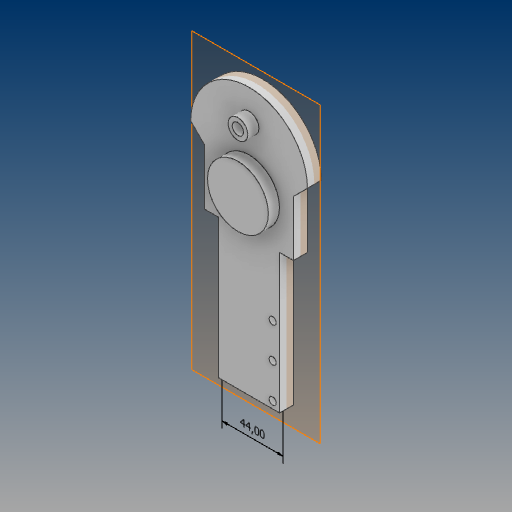
# Autodesk Inventor part: 17_Khau_noi_tiep_cuoi
Saved by Autodesk Inventor 2021 (Build 250183000, 183)
## iProperties
Created: 2024-04-05
Part Number: 17_Khau_noi_tiep_cuoi
Material: Generic
Document SubType Name: Modeling
Designer: Admin
Density: 1 g/cm^3
Appearance: Default
Author: Admin
Autodesk Inventor part; units mm, degrees
ref_plane "YZ Plane" through (0, 0, 0) normal (1, 0, 0) x (0, 1, 0)
ref_plane "XZ Plane" through (0, 0, 0) normal (0, 1, 0) x (-1, 0, 0)
ref_plane "XY Plane" through (0, 0, 0) normal (0, 0, 1) x (1, 0, 0)
sketch "Sketch1" plane through (0, 0, 0) normal (0, 0, 1) x (1, 0, 0)
  arc A0 (-44.1071, -48.8952) -> (-20.8929, -67.8977) centre (-32.5, -58.3964) ccw projected
  arc A1 (-43.869, -48.6061) -> (-44.1071, -48.8952) centre (0, -85) ccw projected
  line L0 (-36.9673, -34.403) -> (-43.869, -48.6061) projected
  arc A2 (-36.9673, -34.403) -> (-25, 17.6067) centre (-144, 17.6067) ccw projected
  line L1 (-25, 17.6067) -> (-25, 75) projected
  line L2 (-25, 75) -> (25, 75) projected
  line L3 (25, 75) -> (25, 17.6067) projected
  arc A3 (25, 17.6067) -> (36.9673, -34.403) centre (144, 17.6067) ccw projected
  line L4 (43.869, -48.6061) -> (36.9673, -34.403) projected
  arc A4 (44.1071, -48.8952) -> (43.869, -48.6061) centre (0, -85) ccw projected
  arc A5 (20.8929, -67.8977) -> (44.1071, -48.8952) centre (32.5, -58.3964) ccw projected
  arc A6 (20.8929, -67.8977) -> (-20.8929, -67.8977) centre (0, -85) ccw projected
  circle A7 centre (-16, 24) radius 2.1 projected
  circle A8 centre (16, 60) radius 2.1 projected
  circle A9 centre (-16, 60) radius 2.1 projected
  circle A10 centre (16, 24) radius 2.1 projected
  arc A11 (38.0714, -53.8358) -> (-38.0714, -53.8358) centre (0, -85) ccw projected
  arc A12 (-38.0714, -53.8358) -> (-26.9286, -62.957) centre (-32.5, -58.3964) ccw projected
  arc A13 (26.9286, -62.957) -> (-26.9286, -62.957) centre (0, -85) ccw projected
  arc A14 (26.9286, -62.957) -> (38.0714, -53.8358) centre (32.5, -58.3964) ccw projected
  circle A15 centre (0, -43) radius 7.1
  line L5 (0, -35.8) -> (0, -50.2) construction
  circle A16 centre (0, -85) radius 21.9
  line L6 (0, -63) -> (0, -213) construction
  line L7 (-42, -63) -> (-42, -213)
  line L8 (42, -213) -> (42, -63)
  arc A17 (42, -63) -> (-42, -63) centre (0, -63) ccw
  arc A18 (-42, -213) -> (42, -213) centre (0, -213) ccw
  point P0 (0, 0)
  point P1 (0, -138)
  dimension "d0" = 14.2
  dimension "d1" = 7.2
  dimension "d2" = 27
  dimension "d3" = 43.8
  dimension "d4" = 42
  dimension "d5" = 150
  dimension "d6" = 20
  constraints: 10 end point, 6 point on circle, 4 centre point, 4 tangent, 2 midpoint, 1 coincident, 1 parallel, 1 vertical, 1 vertical alignment
  measures "d0" diameter of A15
  measures "d1" radius of A12
  measures "d2" radius of A6
  measures "d3" diameter of A16
  measures "d4" radius of A18
  measures "d5" distance of L6.start L6.end
  measures "d6" distance of L6.start A15.centre
extrude "Extrusion1" add sketch "Sketch1" against normal blind 8 contours A15 | A16
sketch "Sketch2" plane through (0, -85, 0) normal (0, 0, 1) x (1, 0, 0)
  line L0 (-42, 22) -> (-42, -128) projected
  arc A0 (42, 22) -> (-42, 22) centre (0, 22) ccw projected
  line L1 (42, -128) -> (42, 22) projected
  arc A1 (-42, -128) -> (42, -128) centre (0, -128) ccw projected
  circle A2 centre (0, 0) radius 21.9 projected
  circle A3 centre (0, 42) radius 7.1 projected
  point P0 (0, 85)
extrude "Extrusion2" add sketch "Sketch2" along normal blind 10 contours A0 L1 A1 L0 | A2 | A3
sketch "Sketch4" plane through (0, -85, 0) normal (0, 0, -1) x (-1, 0, 0)
  circle A0 centre (0, 0) radius 21.9 projected
  circle A1 centre (0, 42) radius 7.1 projected
  arc A2 (-42, -128) -> (42, -128) centre (0, -128) ccw projected
  line L0 (42, 22) -> (42, -128) projected
  arc A3 (42, 22) -> (-42, 22) centre (0, 22) ccw projected
  line L1 (-42, -128) -> (-42, 22) projected
  arc A4 (-42, -128) -> (42, -128) centre (0, -128) ccw projected
  line L2 (42, -128) -> (-42, -128)
  line L3 (32, -128) -> (32, 12)
  arc A5 (42, 22) -> (-42, 22) centre (0, 22) ccw projected
  line L4 (32, 12) -> (42, 22)
  line L5 (0, -128) -> (0, 42) construction
  line L6 (-32, -128) -> (-32, 12)
  line L7 (-32, 12) -> (-42, 22)
  line L8 (22, -128) -> (22, -28)
  line L9 (22, -28) -> (32, -28)
  line L10 (-22, -128) -> (-22, -28)
  line L11 (-22, -28) -> (-32, -28)
  point P0 (0, 85)
  point P1 (-32, -28)
  dimension "d18" = 10
  dimension "d19" = 135
  dimension "d22" = 10
  dimension "d23" = 100
  constraints: 20 end point, 5 symmetric about line, 3 point on line, 2 perpendicular, 2 vertical, 1 horizontal
  measures "d18" distance between parallel lines of L0 L3
  measures "d19" angle of L3 L4
  measures "d22" distance between parallel lines of L3 L8
  measures "d23" distance between parallel lines of L2 L9
extrude "Extrusion3" cut sketch "Sketch4" against normal blind 10 contours L2 A2 | L1 L7 L6 L2 | L2 L3 L4 L0 | L6 L11 L10 L2 | L2 L8 L9 L3
sketch "Sketch5" plane through (0, -85, 10) normal (0, 0, 1) x (1, 0, 0)
  circle A0 centre (17, -73) radius 2.6 projected
  circle A1 centre (17, -98) radius 2.6 projected
  circle A2 centre (17, -123) radius 2.6 projected
  point P0 (0, 85)
extrude "Extrusion4" cut sketch "Sketch5" against normal through all
ref_plane "Work Plane1" through (0, -85, 5) normal (0, 0, 1) x (1, 0, 0)
mirror "Mirror1" about plane through (0, -85, 5) normal (0, 0, 1) of "Extrusion1"
sketch "Sketch3" plane through (0, -43, -8) normal (0, 0, -1) x (-1, 0, 0)
  circle A0 centre (0, 0) radius 7.1 projected
  point P0 (0, 43)
hole "Hole1" at (0, -43, -8) direction (0, 0, 1) diameter 8.2 end through all
body "Solid1"
